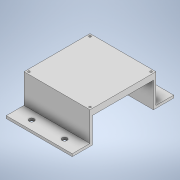
# Autodesk Inventor part: TurntableBase2
Saved by Autodesk Inventor 2020 (Build 240168000, 168)
## iProperties
Created: 2022-02-25
Part Number: TurntableBase2
Material: Generic
Document SubType Name: Modeling
Designer: danie
Density: 1 g/cm^3
Appearance: Default
Author: danie
Autodesk Inventor part; units mm, degrees
ref_plane "YZ Plane" through (0, 0, 0) normal (1, 0, 0) x (0, 1, 0)
ref_plane "XZ Plane" through (0, 0, 0) normal (0, 1, 0) x (-1, 0, 0)
ref_plane "XY Plane" through (0, 0, 0) normal (0, 0, 1) x (1, 0, 0)
sketch "Sketch1" plane through (0, 0, 0) normal (0, 1, 0) x (-1, 0, 0)
  line L0 (0, 0) -> (-82.55, 0)
  line L1 (-82.55, 0) -> (-82.55, -82.55)
  line L2 (-82.55, -82.55) -> (0, -82.55)
  line L3 (0, -82.55) -> (0, 0)
  dimension "d0" = 82.55
  dimension "d1" = 82.55
  constraints: 8 end point, 2 parallel, 1 horizontal, 1 perpendicular
  measures "d0" distance of L2.end L1.end
  measures "d1" distance of L1.end L0.end
extrude "Extrusion1" add sketch "Sketch1" along normal blind 7.62
sketch "Sketch2" plane through (0, 0, 0) normal (0, -1, 0) x (1, 0, 0)
  line L0 (82.55, 0) -> (82.55, -82.55) projected
  line L1 (82.55, 0) -> (0, 0)
  line L2 (0, 0) -> (0, -3.175)
  line L3 (0, -3.175) -> (82.55, -3.175)
  line L4 (82.55, -3.175) -> (82.55, 0)
  line L5 (82.55, -82.55) -> (0, -82.55)
  line L6 (0, -82.55) -> (0, -79.375)
  line L7 (0, -79.375) -> (82.55, -79.375)
  line L8 (82.55, -79.375) -> (82.55, -82.55)
  dimension "d4" = 82.55
  dimension "d5" = 3.175
  dimension "d6" = 82.55
  dimension "d7" = 3.175
  constraints: 16 end point, 4 parallel, 2 horizontal, 2 perpendicular
  measures "d4" distance of L3.end L2.end
  measures "d5" distance of L2.end L1.end
  measures "d6" distance of L6.end L7.end
  measures "d7" distance of L5.end L6.end
extrude "Extrusion2" add sketch "Sketch2" along normal blind 32.0802
sketch "Sketch3" plane through (0, 7.62, 0) normal (0, 1, 0) x (1, 0, 0)
  line L0 (0, 82.55) -> (82.55, 82.55) construction
  line L1 (0, 0) -> (82.55, 82.55) construction
  line L2 (82.55, 0) -> (0, 0) construction
  line L3 (0, 82.55) -> (82.55, 0) construction
  circle A0 centre (3.0661, 3.0077) radius 1.27
  circle A1 centre (3.0661, 79.5423) radius 1.27
  circle A2 centre (79.4839, 79.5423) radius 1.27
  circle A3 centre (79.4839, 3.0077) radius 1.27
  line L4 (3.0661, 3.0077) -> (79.4839, 79.5423) construction
  line L5 (3.0661, 79.5423) -> (79.4839, 3.0077) construction
  dimension "d14" = 2.54
  dimension "d15" = 2.54
  dimension "d16" = 2.54
  dimension "d17" = 2.54
  constraints: 8 end point, 4 centre point
  measures "d14" diameter of A0
  measures "d15" diameter of A1
  measures "d16" diameter of A2
  measures "d17" diameter of A3
extrude "Extrusion3" cut sketch "Sketch3" against normal blind 7.366
sketch "Sketch4" plane through (82.55, 7.62, -82.55) normal (0, 0, -1) x (-1, 0, 0)
  line L0 (0, 0) -> (0, -39.7002) projected
  line L1 (0, -39.7002) -> (82.55, -39.7002)
  line L2 (82.55, -39.7002) -> (82.55, -36.5252)
  line L3 (82.55, -36.5252) -> (0, -36.5252)
  line L4 (0, -36.5252) -> (0, -39.7002)
  point P0 (82.55, -7.62)
  dimension "d20" = 82.55
  dimension "d21" = 3.175
  constraints: 8 end point, 2 parallel, 1 horizontal, 1 perpendicular
  measures "d20" distance of L3.end L2.end
  measures "d21" distance of L2.end L1.end
extrude "Extrusion4" add sketch "Sketch4" along normal blind 22.225
sketch "Sketch5" plane through (0, 7.62, 0) normal (0, 0, 1) x (1, 0, 0)
  line L0 (82.55, -39.7002) -> (0, -39.7002) projected
  line L1 (0, -39.7002) -> (82.55, -39.7002)
  line L2 (82.55, -39.7002) -> (82.55, -36.5252)
  line L3 (82.55, -36.5252) -> (0, -36.5252)
  line L4 (0, -36.5252) -> (0, -39.7002)
  point P0 (0, -7.62)
  dimension "d24" = 82.55
  dimension "d25" = 3.175
  constraints: 8 end point, 2 parallel, 1 horizontal, 1 perpendicular
  measures "d24" distance of L3.end L2.end
  measures "d25" distance of L2.end L1.end
extrude "Extrusion5" add sketch "Sketch5" along normal blind 22.225
sketch "Sketch6" plane through (0, -28.9052, 0) normal (0, 1, 0) x (1, 0, 0)
  line L0 (0, 0) -> (0, -22.225) construction
  line L1 (0, -22.225) -> (0, -11.1125) construction
  line L2 (0, -11.1125) -> (20.6375, -11.1125) construction
  line L3 (20.6375, -11.1125) -> (61.9125, -11.1125) construction
  line L4 (0, 79.375) -> (0, 104.775) construction
  line L5 (0, 104.775) -> (0, 93.6625) construction
  line L6 (0, 93.6625) -> (20.6375, 93.6625) construction
  line L7 (20.6375, 93.6625) -> (61.9125, 93.6625) construction
  circle A0 centre (20.6375, -11.1125) radius 3.175
  circle A1 centre (20.6375, 93.6625) radius 3.175
  circle A2 centre (61.9125, 93.6625) radius 3.175
  circle A3 centre (61.9125, -11.1125) radius 3.175
  dimension "d28" = 11.1125
  dimension "d29" = 20.6375
  dimension "d30" = 41.275
  dimension "d31" = 11.1125
  dimension "d32" = 20.6375
  dimension "d33" = 90
  dimension "d34" = 41.275
  dimension "d35" = 180
  dimension "d36" = 6.35
  dimension "d37" = 6.35
  dimension "d38" = 6.35
  dimension "d39" = 6.35
  constraints: 12 end point, 4 centre point, 4 coincident, 2 point on line, 1 collinear, 1 horizontal, 1 midpoint, 1 perpendicular
  measures "d28" distance of L0.end L1.end
  measures "d29" distance of L1.end L2.end
  measures "d30" distance of L2.end L3.end
  measures "d31" distance of L4.end L5.end
  measures "d32" distance of L5.end L6.end
  measures "d33" angle of L6 L5
  measures "d34" distance of L6.end L7.end
  measures "d35" angle of L7 L6
  measures "d36" diameter of A0
  measures "d37" diameter of A1
  measures "d38" diameter of A2
  measures "d39" diameter of A3
extrude "Extrusion6" cut sketch "Sketch6" against normal blind 3.175
body "Solid1"
